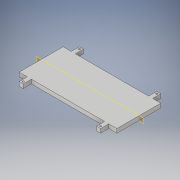
# Autodesk Inventor part: BottomPanel
Saved by Autodesk Inventor 2018 (Build 220112000, 112)
## iProperties
Created: 2018-10-20
Part Number: BottomPanel
Material: Generic
Document SubType Name: Modeling
Designer: jpark
Density: 1 g/cm^3
Appearance: Default
Author: jpark
Autodesk Inventor part; units mm, degrees
ref_plane "YZ Plane" through (0, 0, 0) normal (1, 0, 0) x (0, 1, 0)
ref_plane "XZ Plane" through (0, 0, 0) normal (0, 1, 0) x (-1, 0, 0)
ref_plane "XY Plane" through (0, 0, 0) normal (0, 0, 1) x (1, 0, 0)
sketch "Sketch1" plane through (0, 0, 0) normal (0, 1, 0) x (-1, 0, 0)
  line L0 (0, 0) -> (152.4, 0)
  line L1 (152.4, 0) -> (152.4, -68.58)
  line L2 (152.4, -68.58) -> (0, -68.58)
  line L3 (0, -68.58) -> (0, 0)
  dimension "d0" = 152.4
  dimension "d1" = 68.58
  constraints: 8 end point, 2 parallel, 1 horizontal, 1 perpendicular
  measures "d0" distance of L1.end L2.end
  measures "d1" distance of L0.end L1.end
extrude "Extrusion1" add sketch "Sketch1" along normal blind 6.35
sketch "Sketch2" plane through (0, 6.35, 0) normal (0, 1, 0) x (1, 0, 0)
  line L0 (-133.35, 0) -> (-139.7, 0)
  line L1 (-139.7, 0) -> (-139.7, -12.7)
  line L2 (-139.7, -12.7) -> (-133.35, -12.7)
  line L3 (-133.35, -12.7) -> (-133.35, 0)
  circle A0 centre (-136.525, -9.525) radius 1.397
  line L4 (-152.4, 0) -> (0, 0) projected
  line L5 (-12.7, 0) -> (-19.05, 0)
  line L6 (-19.05, 0) -> (-19.05, -12.7)
  line L7 (-19.05, -12.7) -> (-12.7, -12.7)
  line L8 (-12.7, -12.7) -> (-12.7, 0)
  circle A1 centre (-15.875, -9.525) radius 1.397
  dimension "d4" = 12.7
  dimension "d5" = 6.35
  dimension "d6" = 2.794
  dimension "d7" = 3.175
  dimension "d8" = 3.175
  dimension "d9" = 0
  dimension "d10" = 12.7
  dimension "d11" = 12.7
  dimension "d12" = 6.35
  dimension "d13" = 2.794
  dimension "d14" = 3.175
  dimension "d15" = 3.175
  dimension "d16" = 0
  dimension "d17" = 12.7
  constraints: 16 end point, 4 parallel, 2 centre point, 2 horizontal, 2 perpendicular
  measures "d4" distance of L0.end L1.end
  measures "d5" distance of L1.end L2.end
  measures "d6" diameter of A0
  measures "d7" distance from line of L2 A0.centre
  measures "d8" distance from line of L3 A0.centre
  measures "d9" distance between parallel lines of L4 L0
  measures "d10" distance from line of L4.start L1
  measures "d11" distance of L5.end L6.end
  measures "d12" distance of L6.end L7.end
  measures "d13" diameter of A1
  measures "d14" distance from line of L7 A1.centre
  measures "d15" distance from line of L8 A1.centre
  measures "d16" distance between parallel lines of L4 L5
  measures "d17" distance from line of L4.end L8
extrude "Extrusion2" add sketch "Sketch2" against normal blind 6.35
ref_plane "Work Plane1" through (-133.35, 0, -34.29) normal (0, 0, 1) x (1, 0, 0)
mirror "Mirror1" about plane through (-133.35, 0, -34.29) normal (0, 0, 1) of "Extrusion2"
body "Solid1"
